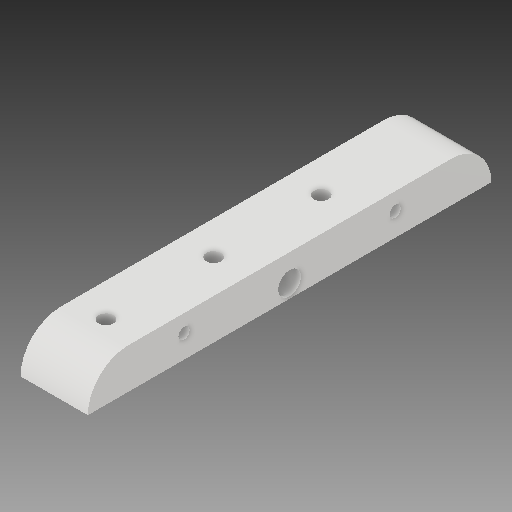
# Autodesk Inventor part: Plastic Holders
Saved by Autodesk Inventor 2019.4 (Build 234330000, 330)
## iProperties
Created: 2019-12-14
Part Number: Plastic Holders
Material: PC/ABS Plastic
Document SubType Name: Modeling
Designer: Mark
Density: 0.357273 g/cm^3
Appearance: Smooth - White
Author: Mark
Autodesk Inventor part; units mm, degrees
ref_plane "YZ Plane" through (0, 0, 0) normal (1, 0, 0) x (0, 1, 0)
ref_plane "XZ Plane" through (0, 0, 0) normal (0, 1, 0) x (-1, 0, 0)
ref_plane "XY Plane" through (0, 0, 0) normal (0, 0, 1) x (1, 0, 0)
sketch "Sketch1" plane through (0, 0, 0) normal (1, 0, 0) x (0, 1, 0)
  line L0 (-7.5, 75) -> (7.5, 75)
  line L1 (7.5, 75) -> (7.5, -75)
  line L2 (7.5, -75) -> (-7.5, -75)
  line L3 (-7.5, -75) -> (-7.5, 75)
  line L4 (-7.5, 75) -> (7.5, -75) construction
  line L5 (7.5, 75) -> (-7.5, -75) construction
  point P0 (0, 0)
  dimension "d0" = 15
  dimension "d1" = 150
  constraints: 12 end point, 2 midpoint, 2 parallel, 1 horizontal, 1 perpendicular
  measures "d0" distance of L1.end L2.end
  measures "d1" distance of L0.end L1.end
extrude "Extrusion1" add sketch "Sketch1" along normal blind 25
sketch "Sketch2" plane through (25, 0, 0) normal (1, 0, 0) x (0, 0, -1)
  circle A0 centre (-39.23, 1) radius 2.1
  circle A1 centre (39.23, 1) radius 2.1
  line L0 (-75, -7.5) -> (75, -7.5) projected
  line L1 (-75, 7.5) -> (-75, -7.5) projected
  line L2 (75, -7.5) -> (75, 7.5) projected
  point P0 (0, 0)
  dimension "d4" = 4.2
  dimension "d5" = 4.2
  dimension "d6" = 8.5
  dimension "d7" = 78.46
  dimension "d8" = 35.77
  dimension "d9" = 8.5
  dimension "d10" = 35.77
  constraints: 2 centre point
  measures "d4" diameter of A0
  measures "d5" diameter of A1
  measures "d6" distance from line of L0 A0.centre
  measures "d7" distance of A1.centre A0.centre
  measures "d8" distance from line of L1 A0.centre
  measures "d9" distance from line of L0 A1.centre
  measures "d10" distance from line of L2 A1.centre
extrude "Extrusion2" cut sketch "Sketch2" against normal blind 25
fillet "Fillet1" radius 15 2 edges at (12.5, 7.5, 75) (12.5, 7.5, -75)
sketch "Sketch3" plane through (25, 0, 0) normal (1, 0, 0) x (0, 0, -1)
  circle A0 centre (0, -2.5) radius 4.25
  line L0 (60, 7.5) -> (-60, 7.5) projected
  arc A1 (75, -7.5) -> (60, 7.5) centre (60, -7.5) ccw projected
  point P0 (0, 0)
  dimension "d14" = 8.5
  dimension "d15" = 10
  dimension "d16" = 60
  constraints: 1 centre point
  measures "d14" diameter of A0
  measures "d15" distance from line of L0 A0.centre
  measures "d16" horizontal distance of A1.centre A0.centre
extrude "Extrusion3" cut sketch "Sketch3" against normal blind 25
sketch "Sketch4" plane through (0, 7.5, 60) normal (0, 1, 0) x (1, 0, 0)
  circle A0 centre (12.5, 4.23) radius 2.75 projected
  circle A1 centre (12.5, 44.23) radius 2.75 projected
  circle A2 centre (12.5, 84.23) radius 2.75 projected
  point P0 (0, 60)
extrude "Extrusion4" cut sketch "Sketch4" against normal blind 25
body "Solid1"
